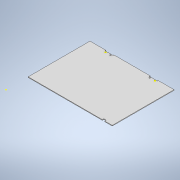
# Autodesk Inventor part: 220207 Lid
Saved by Autodesk Inventor 2022 (Build 260153000, 153)
## iProperties
Created: 2022-02-07
Part Number: 220207 Lid
Material: Generic
Document SubType Name: Modeling
Designer: josephinew
Density: 1 g/cm^3
Appearance: Default
Author: josephinew
Autodesk Inventor part; units mm, degrees
ref_plane "YZ Plane" through (0, 0, 0) normal (1, 0, 0) x (0, 1, 0)
ref_plane "XZ Plane" through (0, 0, 0) normal (0, 1, 0) x (-1, 0, 0)
ref_plane "XY Plane" through (0, 0, 0) normal (0, 0, 1) x (1, 0, 0)
sketch "Sketch1" plane through (0, 0, 0) normal (0, 1, 0) x (-1, 0, 0)
  line L0 (0, 0) -> (-431.8, 0)
  line L1 (-431.8, 0) -> (-431.8, -431.8)
  line L2 (-431.8, -431.8) -> (0, -431.8)
  line L3 (0, -431.8) -> (0, 0)
  dimension "d0" = 431.8
  dimension "d1" = 431.8
  constraints: 8 end point, 2 parallel, 1 horizontal, 1 perpendicular
  measures "d0" distance of L2.end L1.end
  measures "d1" distance of L1.end L0.end
extrude "Extrusion1" add sketch "Sketch1" along normal blind 3.175
sketch "Sketch2" plane through (0, 3.175, 0) normal (0, 1, 0) x (1, 0, 0)
  line L0 (0, 431.8) -> (0, 0) projected
  line L1 (431.8, 0) -> (431.8, 431.8) projected
  circle A0 centre (386.08, 64.77) radius 6.35
  circle A1 centre (332.74, 64.77) radius 6.35
  circle A2 centre (279.4, 64.77) radius 6.35
  circle A3 centre (226.06, 64.77) radius 6.35
  circle A4 centre (172.72, 64.77) radius 6.35
  circle A5 centre (28.43, 92.2674) radius 1.5
  circle A6 centre (121.43, 92.2674) radius 1.5
  circle A7 centre (28.43, 37.2726) radius 1.5
  circle A8 centre (121.43, 37.2726) radius 1.5
  line L2 (26.43, 84.77) -> (123.43, 84.77)
  line L3 (123.43, 84.77) -> (123.43, 44.77)
  line L4 (123.43, 44.77) -> (26.43, 44.77)
  line L5 (26.43, 44.77) -> (26.43, 84.77)
  dimension "d14" = 12.7
  dimension "d15" = 12.7
  dimension "d16" = 12.7
  dimension "d17" = 12.7
  dimension "d18" = 12.7
  constraints: 9 centre point, 8 end point, 2 parallel, 1 horizontal, 1 perpendicular
  measures "d14" diameter of A0
  measures "d15" diameter of A1
  measures "d16" diameter of A2
  measures "d17" diameter of A3
  measures "d18" diameter of A4
extrude "Extrusion2" cut sketch "Sketch2" against normal blind 25.4
sketch "Sketch3" plane through (0, 3.175, 0) normal (0, 1, 0) x (1, 0, 0)
  circle A0 centre (88.9, 421.64) radius 2.794
  circle A1 centre (115.316, 421.64) radius 2.794
  circle A2 centre (316.484, 421.64) radius 2.794
  circle A3 centre (342.9, 421.64) radius 2.794
  line L0 (0, 431.8) -> (0, 0) projected
  line L1 (431.8, 0) -> (431.8, 431.8) projected
  constraints: 4 centre point
extrude "Extrusion3" cut sketch "Sketch3" along normal blind 25.4 and the other way blind 12.7
sketch "Sketch4" plane through (0, 0, 0) normal (0, -1, 0) x (1, 0, 0)
  circle A0 centre (386.08, -64.77) radius 6.35 projected
  circle A1 centre (386.08, -64.77) radius 7.62
  circle A2 centre (172.72, -64.77) radius 6.35 projected
  circle A3 centre (172.72, -64.77) radius 7.62
  circle A4 centre (226.06, -64.77) radius 6.35 projected
  circle A5 centre (226.06, -64.77) radius 7.62
  circle A6 centre (279.4, -64.77) radius 6.35 projected
  circle A7 centre (279.4, -64.77) radius 7.62
  circle A8 centre (332.74, -64.77) radius 6.35 projected
  circle A9 centre (332.74, -64.77) radius 7.62
  point P0 (0, 0)
  dimension "d50" = 15.24
  dimension "d51" = 15.24
  dimension "d52" = 15.24
  dimension "d53" = 15.24
  dimension "d54" = 15.24
  constraints: 5 centre point, 5 coincident
  measures "d50" diameter of A1
  measures "d51" diameter of A3
  measures "d52" diameter of A5
  measures "d53" diameter of A7
  measures "d54" diameter of A9
extrude "Extrusion4" cut sketch "Sketch4" against normal blind 4.351 contours A0 | A1 | A2 | A3 | A4 | A5 | A6 | A7 | A8 | A9
sketch "Sketch5" plane through (0, 3.175, 0) normal (0, 1, 0) x (1, 0, 0)
  line L0 (0, 431.8) -> (431.8, 431.8)
  line L1 (431.8, 431.8) -> (431.8, 114.3)
  line L2 (431.8, 114.3) -> (0, 114.3)
  line L3 (0, 114.3) -> (0, 431.8)
  line L4 (0, 114.3) -> (431.8, 114.3)
  line L5 (0, -12.7) -> (0, 114.3)
  line L6 (0, -12.7) -> (0, 0)
  line L7 (431.8, 0) -> (431.8, 431.8) projected
  line L8 (0, 114.3) -> (431.8, 114.3)
  line L9 (431.8, 114.3) -> (431.8, 12.7)
  line L10 (431.8, 12.7) -> (0, 12.7)
  line L11 (0, 12.7) -> (0, 114.3)
  line L12 (0, 12.7) -> (431.8, 12.7)
  line L13 (431.8, 12.7) -> (431.8, 0)
  line L14 (431.8, 0) -> (0, 0)
  line L15 (0, 0) -> (0, 12.7)
  dimension "d57" = 317.5
  dimension "d59" = 101.6
  constraints: 30 end point, 6 parallel, 4 horizontal, 3 perpendicular, 1 point on line
  measures "d57" distance of L0.end L1.end
  measures "d59" distance of L8.end L9.end
extrude "Extrusion5" cut sketch "Sketch5" against normal blind 25.4 contours L2 L7 L10 L5 | L10 L7 L14 L5
sketch "Sketch7" plane through (0, 3.175, 0) normal (0, 1, 0) x (1, 0, 0)
  line L0 (431.8, 114.3) -> (431.8, 431.8) projected
  line L1 (393.7, 114.3) -> (381, 114.3)
  line L2 (381, 114.3) -> (381, 121.92)
  line L3 (381, 121.92) -> (393.7, 121.92)
  line L4 (393.7, 121.92) -> (393.7, 114.3)
  point P0 (0, 0)
  dimension "d63" = 12.7
  dimension "d64" = 7.62
  constraints: 8 end point, 2 parallel, 1 horizontal, 1 perpendicular
  measures "d63" distance of L2.end L3.end
  measures "d64" distance of L1.end L2.end
extrude "Extrusion6" cut sketch "Sketch7" against normal blind 25.4
sketch "Sketch8" plane through (0, 3.175, 0) normal (0, 1, 0) x (1, 0, 0)
  point P0 (0, 0)
sketch "Sketch9" plane through (0, 3.175, 0) normal (0, 1, 0) x (1, 0, 0)
  circle A0 centre (88.9, 421.64) radius 2.794 projected
  circle A1 centre (342.9, 421.64) radius 2.794 projected
  point P0 (0, 0)
sketch "Sketch10" plane through (0, 3.175, 0) normal (0, 1, 0) x (1, 0, 0)
  circle A0 centre (115.316, 421.64) radius 2.794 projected
  line L0 (115.316, 421.64) -> (121.158, 421.64)
  line L1 (121.158, 421.64) -> (121.158, 431.8)
  line L2 (431.8, 431.8) -> (0, 431.8) projected
  line L3 (121.158, 431.8) -> (83.058, 431.8)
  line L4 (83.058, 431.8) -> (83.058, 421.64)
  circle A1 centre (88.9, 421.64) radius 2.794 projected
  line L5 (83.058, 421.64) -> (88.9, 421.64)
  circle A2 centre (342.9, 421.64) radius 2.794 projected
  line L6 (342.9, 421.64) -> (348.742, 421.64)
  line L7 (348.742, 421.64) -> (348.742, 431.8)
  line L8 (348.742, 431.8) -> (310.642, 431.8)
  line L9 (310.642, 431.8) -> (310.642, 421.64)
  circle A3 centre (316.484, 421.64) radius 2.794 projected
  line L10 (310.642, 421.64) -> (316.484, 421.64)
  line L11 (83.058, 431.8) -> (83.058, 429.26)
  line L12 (83.058, 429.26) -> (121.158, 429.26)
  line L13 (310.642, 431.8) -> (310.642, 429.26)
  line L14 (310.642, 429.26) -> (348.742, 429.26)
  point P0 (0, 0)
  dimension "d73" = 5.842
  dimension "d74" = 38.1
  dimension "d75" = 5.842
  dimension "d76" = 38.1
  dimension "d77" = 2.54
  dimension "d78" = 2.54
  constraints: 28 end point, 9 perpendicular, 9 point on line, 2 horizontal
  measures "d73" distance of L0.start L0.end
  measures "d74" distance of L1.end L3.end
  measures "d75" distance of L6.start L6.end
  measures "d76" distance of L7.end L8.end
  measures "d77" distance of L3.end L11.end
  measures "d78" distance of L8.end L13.end
extrude "Extrusion7" cut sketch "Sketch10" against normal blind 25.4 contours L2 L7 L14 L9 | L12 L4 L2 L1
sketch "Sketch12" plane through (0, 3.175, 0) normal (0, 1, 0) x (1, 0, 0)
  line L0 (102.108, 431.8) -> (122.7455, 431.8)
  line L1 (310.642, 431.8) -> (121.158, 431.8) projected
  line L2 (102.108, 431.8) -> (81.4705, 431.8)
  line L3 (81.4705, 431.8) -> (81.4705, 429.26)
  line L4 (121.158, 429.26) -> (83.058, 429.26) projected
  line L5 (122.7455, 429.26) -> (122.7455, 431.8)
  line L6 (121.158, 429.26) -> (121.158, 431.8)
  line L7 (83.058, 431.8) -> (0, 431.8) projected
  line L8 (81.4705, 431.8) -> (81.4705, 427.4312)
  line L9 (81.4705, 427.4312) -> (122.7455, 427.4312)
  line L10 (122.7455, 427.4312) -> (122.7455, 429.26)
  line L11 (83.058, 429.26) -> (83.058, 427.4312)
  line L12 (121.158, 429.26) -> (121.158, 427.4312)
  line L13 (431.8, 431.8) -> (348.742, 431.8) projected
  line L14 (348.742, 431.8) -> (348.742, 434.6291)
  line L15 (329.692, 431.8) -> (350.3295, 431.8)
  line L16 (329.692, 431.8) -> (309.0545, 431.8)
  line L17 (309.0545, 431.8) -> (309.0545, 429.26)
  line L18 (350.3295, 429.26) -> (350.3295, 431.8)
  line L19 (348.742, 429.26) -> (348.742, 431.8)
  line L20 (309.0545, 431.8) -> (309.0545, 427.4312)
  line L21 (309.0545, 427.4312) -> (350.3295, 427.4312)
  line L22 (350.3295, 427.4312) -> (350.3295, 429.26)
  line L23 (310.642, 429.26) -> (310.642, 427.4312)
  line L24 (348.742, 429.26) -> (348.742, 427.4312)
  point P0 (0, 0)
  dimension "d84" = 20.6375
  dimension "d87" = 4.3688
  dimension "d89" = 4.3688
  constraints: 42 end point, 11 perpendicular, 5 point on line, 5 vertical, 2 horizontal
  measures "d84" distance of L0.start L0.end
  measures "d87" distance of L2.end L8.end
  measures "d89" distance of L17.start L20.end
extrude "Extrusion8" cut sketch "Sketch12" against normal blind 25.4
body "Solid1"
